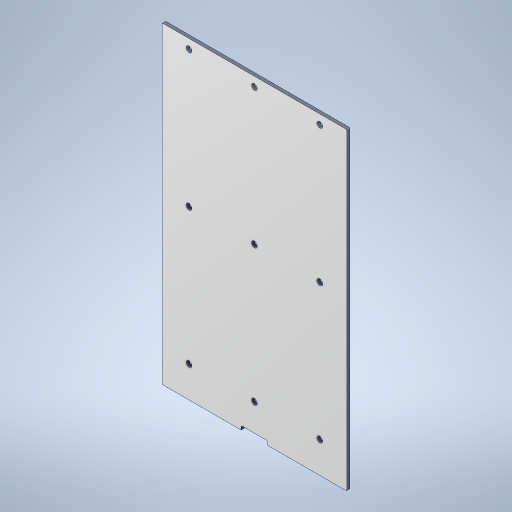
# Autodesk Inventor part: Medium Internal Vertical Side Panels
Saved by Autodesk Inventor 2024 (Build 280153000, 153)
## iProperties
Created: 2024-09-28
Part Number: Medium Internal Vertical Side Panels
Material: Generic
Document SubType Name: Modeling
Designer: Ishaan
Density: 1 g/cm^3
Appearance: Default
Author: Ishaan
Autodesk Inventor part; units mm, degrees
ref_plane "YZ Plane" through (0, 0, 0) normal (1, 0, 0) x (0, 1, 0)
ref_plane "XZ Plane" through (0, 0, 0) normal (0, 1, 0) x (-1, 0, 0)
ref_plane "XY Plane" through (0, 0, 0) normal (0, 0, 1) x (1, 0, 0)
sketch "Sketch1" plane through (0, 0, 0) normal (0, 0, 1) x (1, 0, 0)
  line L0 (84.75, -143.625) -> (-84.75, -143.625)
  line L1 (-84.75, -143.625) -> (-84.75, 143.625)
  line L2 (-84.75, 143.625) -> (84.75, 143.625)
  line L3 (84.75, 143.625) -> (84.75, -143.625)
  line L4 (84.75, -143.625) -> (-84.75, 143.625) construction
  line L5 (-84.75, -143.625) -> (84.75, 143.625) construction
  point P0 (0, 0)
  dimension "d0" = 169.5
  dimension "d1" = 287.25
  constraints: 12 end point, 2 midpoint, 2 parallel, 1 horizontal, 1 perpendicular
  measures "d0" distance of L1.end L2.end
  measures "d1" distance of L0.end L1.end
extrude "Extrusion1" add sketch "Sketch1" along normal mid plane 3
extrude "Extrusion2" cut sketch "Sketch1" along normal mid plane 2.9
extrude "Extrusion3" add sketch "Sketch1" along normal mid plane 2.9 separate body
sketch "Sketch2" plane through (0, 0, 1.5) normal (0, 0, 1) x (1, 0, 0)
  line L0 (-84.75, -143.625) -> (84.75, -143.625) projected
  line L1 (60, -115) -> (-60, -115) construction
  line L2 (-60, -115) -> (-60, 135) construction
  line L3 (-60, 135) -> (60, 135) construction
  line L4 (60, 135) -> (60, -115) construction
  line L5 (60, -115) -> (-60, 135) construction
  line L6 (-60, -115) -> (60, 135) construction
  point P0 (0, 0)
  point P1 (0, 10)
  point P2 (0, 135)
  point P3 (-60, 10)
  point P4 (60, 10)
  point P5 (0, -115)
  point P6 (60, 10)
  point P7 (0, 10)
  point P8 (-60, 10)
  dimension "d19" = 250
  dimension "d20" = 120
  dimension "d22" = 10
  constraints: 12 end point, 7 coincident, 6 midpoint, 2 parallel, 1 horizontal, 1 perpendicular, 1 vertical alignment
  measures "d19" distance of L1.end L2.end
  measures "d20" distance of L2.end L3.end
  measures "d22" distance of point (0, 10) point (0, 0)
hole "Hole1" at (-60, 135, 1.5) at (-60, 10, 1.5) at (-60, -115, 1.5) at (0, -115, 1.5) at (60, -115, 1.5) at (60, 10, 1.5) at (0, 10, 1.5) at (0, 135, 1.5) at (60, 135, 1.5) direction (0, 0, -1) diameter 5.4 end through all bodies 1 2
sketch "Sketch3" plane through (0, 0, 1.5) normal (0, 0, 1) x (1, 0, 0)
  line L0 (-12, -143.625) -> (12, -143.625)
  line L1 (12, -143.625) -> (12, -141)
  line L2 (11, -140) -> (-11, -140)
  line L3 (-12, -141) -> (-12, -143.625)
  line L4 (-84.75, -143.625) -> (84.75, -143.625) projected
  arc A0 (-11, -140) -> (-12, -141) centre (-11, -141) ccw
  arc A1 (12, -141) -> (11, -140) centre (11, -141) ccw
  point P0 (0, 0)
  point P1 (12, -140)
  point P2 (-12, -140)
  point P3 (0, -143.625)
  dimension "d23" = 24
  dimension "d24" = 3.625
  dimension "d27" = 1
  constraints: 8 end point, 4 point on circle, 4 point on line, 4 tangent, 2 centre point, 2 midpoint, 2 parallel, 1 equal radius, 1 horizontal, 1 perpendicular
  measures "d23" distance of point (-12, -140) point (12, -140)
  measures "d24" distance of point (12, -140) L0.end
  measures "d27" radius of A0
extrude "Extrusion4" cut sketch "Sketch3" against normal through all bodies 1 2
